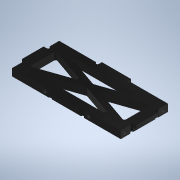
# Autodesk Inventor part: Trunk_horizontal_frame_04
Saved by Autodesk Inventor 2020.4 (Build 244396000, 396)
## iProperties
Created: 2016-05-21
Part Number: Trunk_horizontal_frame_04
Material: アセタール樹脂、黒
Document SubType Name: Modeling
Designer: hiroaki
Density: 1.425 g/cm^3
Appearance: 滑らか - 黒
Mass: 9.76521 g
Surface Area: 55.2384 cm^2
Volume: 6.85278 cm^3
Category: 胴体
d0: 1.050 mm
d1: 32.500 mm
d2: 75.000 mm
d3: 40.000 mm
d48: 26.500 mm
d52: 5.000 mm
d21: 32.500 mm
d23: 2.000 mm
d30: 2.000 mm
d34: 8.750 mm
d53: 20.000 mm
d54: 3.100 mm
d55: 5.000 mm
d56: 5.000 mm
d57: 0.00 deg
d58: 2.500 mm
d59: 0.00 deg
d60: 5.000 mm
d62: 2.500 mm
d66: 2.500 mm
d70: 2.500 mm
d74: 2.500 mm
Author: hiroaki
Autodesk Inventor part; units mm, degrees
ref_plane "YZ Plane" through (0, 0, 0) normal (1, 0, 0) x (0, 1, 0)
ref_plane "XZ Plane" through (0, 0, 0) normal (0, 1, 0) x (-1, 0, 0)
ref_plane "XY Plane" through (0, 0, 0) normal (0, 0, 1) x (1, 0, 0)
sketch "スケッチ1" plane through (0, 0, 0) normal (0, 0, 1) x (1, 0, 0)
  line L0 (-37.5, 9.6) -> (-37.5, 16.25)
  line L1 (-37.5, 16.25) -> (-20, 16.25)
  line L2 (20, 16.25) -> (37.5, 16.25)
  line L3 (37.5, 16.25) -> (37.5, 9.6)
  line L4 (0, 0) -> (0, 16.25) construction
  line L5 (0, 0) -> (39.5, 0) construction
  line L6 (37.5, 7.5) -> (39.5, 7.5)
  line L7 (39.5, 7.5) -> (39.5, -7.5)
  line L8 (39.5, -7.5) -> (37.5, -7.5)
  line L9 (-20, -16.25) -> (20, -16.25) construction
  line L10 (20, -16.25) -> (20, 16.25) construction
  line L11 (20, 16.25) -> (-20, 16.25) construction
  line L12 (-20, 16.25) -> (-20, -16.25) construction
  line L13 (-20, -16.25) -> (20, 16.25) construction
  line L14 (20, -16.25) -> (-20, 16.25) construction
  line L15 (-37.5, -16.25) -> (37.5, -16.25) construction
  line L16 (37.5, -16.25) -> (37.5, 16.25) construction
  line L17 (37.5, 16.25) -> (-37.5, 16.25) construction
  line L18 (-37.5, 16.25) -> (-37.5, -16.25) construction
  line L19 (-37.5, -16.25) -> (37.5, 16.25) construction
  line L20 (37.5, -16.25) -> (-37.5, 16.25) construction
  arc A0 (37.5, 9.6) -> (37.5, 7.5) centre (37.5, 8.55) ccw
  arc A1 (37.5, -7.5) -> (37.5, -9.6) centre (37.5, -8.55) ccw
  line L21 (37.5, -9.6) -> (37.5, -16.25)
  line L22 (37.5, -16.25) -> (20, -16.25)
  line L23 (20, -16.25) -> (12.1, -16.25)
  line L24 (-20, 16.25) -> (-12.1, 16.25)
  line L25 (-10, 16.25) -> (-10, 18.25)
  line L26 (-10, 18.25) -> (10, 18.25)
  line L27 (10, 18.25) -> (10, 16.25)
  line L28 (20, 16.25) -> (12.1, 16.25)
  arc A2 (-12.1, 16.25) -> (-10, 16.25) centre (-11.05, 16.25) ccw
  arc A3 (10, 16.25) -> (12.1, 16.25) centre (11.05, 16.25) ccw
  line L29 (-37.5, 7.5) -> (-39.5, 7.5)
  line L30 (-39.5, 7.5) -> (-39.5, -7.5)
  line L31 (-39.5, -7.5) -> (-37.5, -7.5)
  arc A4 (-37.5, 7.5) -> (-37.5, 9.6) centre (-37.5, 8.55) ccw
  arc A5 (-37.5, -9.6) -> (-37.5, -7.5) centre (-37.5, -8.55) ccw
  line L32 (-37.5, -9.6) -> (-37.5, -16.25)
  line L33 (-37.5, -16.25) -> (-20, -16.25)
  line L34 (-20, -16.25) -> (-12.1, -16.25)
  line L35 (-10, -16.25) -> (-10, -18.25)
  line L36 (-10, -18.25) -> (10, -18.25)
  line L37 (10, -18.25) -> (10, -16.25)
  arc A6 (-10, -16.25) -> (-12.1, -16.25) centre (-11.05, -16.25) ccw
  arc A7 (12.1, -16.25) -> (10, -16.25) centre (11.05, -16.25) ccw
  line L38 (-16.55, 19.1799) -> (-13.45, 19.1799) construction
  line L39 (-13.45, 19.1799) -> (-13.45, 12.4242) construction
  line L40 (-13.45, 12.4242) -> (-16.55, 12.4242) construction
  line L41 (-16.55, 12.4242) -> (-16.55, 19.1799) construction
  line L42 (-15, 19.1799) -> (-15, 12.4242) construction
  point P0 (0, 18.25)
  point P1 (0, 0)
  dimension "d0" = 1.05
  dimension "d1" = 32.5
  dimension "d2" = 75
  dimension "d3" = 40
  dimension "d23" = 2
  dimension "d30" = 2
  dimension "d34" = 8.75
  dimension "d53" = 20
  dimension "d54" = 3.1
  dimension "d55" = 5
  dimension "d85" = 32.5
  constraints: 86 end point, 17 point on line, 16 point on circle, 12 perpendicular, 9 midpoint, 8 centre point, 7 equal radius, 7 parallel, 6 horizontal, 6 symmetric about line, 5 tangent, 4 collinear, 2 vertical, 2 vertical alignment, 1 other
  measures "d0" radius of A0
  measures "d1" distance between parallel lines of L9 L11
  measures "d2" distance of L2.end L0.end
  measures "d3" distance between parallel lines of L10 L12
  measures "d23" distance of L6.start L6.end
  measures "d30" distance between parallel lines of L26 L11
  measures "d34" distance between parallel lines of L17 L29
  measures "d53" distance of L25.end L26.end
  measures "d54" distance of L38.start L38.end
  measures "d55" distance between parallel lines of L25 L42
  measures "d85" distance between parallel lines of L15 L17
extrude "押し出し1" add sketch "スケッチ1" along normal blind 5
sketch "スケッチ2" plane through (0, 0, 0) normal (0, 0, -1) x (-1, 0, 0)
  line L0 (37.5, 9.6) -> (37.5, 16.25) projected
  line L1 (-37.5, 16.25) -> (-37.5, 9.6) projected
  line L2 (-45.6427, 17.3125) -> (-37.5, 17.3125)
  line L3 (-37.5, 17.3125) -> (-37.5, -16.751)
  line L4 (-37.5, -16.751) -> (-45.6427, -16.751)
  line L5 (-45.6427, -16.751) -> (-45.6427, 17.3125)
  line L6 (37.5, 21.1805) -> (43.358, 21.1805)
  line L7 (43.358, 21.1805) -> (43.358, -13.6193)
  line L8 (43.358, -13.6193) -> (37.5, -13.6193)
  line L9 (37.5, -13.6193) -> (37.5, 21.1805)
  line L10 (-20, -16.25) -> (-12.1, -16.25)
  line L11 (-17.1371, 25.1848) -> (11.8342, 25.1848)
  line L12 (11.8342, 25.1848) -> (11.8342, 16.25)
  line L13 (11.8342, 16.25) -> (-17.1371, 16.25)
  line L14 (-17.1371, 16.25) -> (-17.1371, 25.1848)
  line L15 (-13.151, -21.5857) -> (17.7795, -21.5857)
  line L16 (17.7795, -21.5857) -> (17.7795, -16.25)
  line L17 (17.7795, -16.25) -> (-13.151, -16.25)
  line L18 (-13.151, -16.25) -> (-13.151, -21.5857)
  line L19 (-12.1, 16.25) -> (-37.5, 16.25)
  line L20 (-37.5, -16.25) -> (-12.1, -16.25)
  point P0 (0, 0)
  constraints: 38 end point, 8 parallel, 4 horizontal, 4 perpendicular, 3 collinear
extrude "押し出し2" cut sketch "スケッチ2" against normal blind 2.5
sketch "スケッチ3" plane through (12.1, 16.25, 0) normal (0, 1, 0) x (1, 0, 0)
  line L0 (-2.1, 0) -> (-2.1, -5) projected
  line L1 (-2.1, -5) -> (-22.1, -5) construction
  line L2 (-12.1, -5) -> (-12.1, 7.4607) construction
  line L3 (25.4, 0) -> (25.4, -5) projected
  point P0 (-12.1, 0)
  point P1 (2.9, -2.5)
  point P2 (-27.1, -2.5)
  point P3 (25.4, -2.5)
  dimension "d60" = 5
  constraints: 2 end point, 2 horizontal alignment, 2 midpoint, 1 symmetric about line, 1 vertical
  measures "d60" distance from line of L0 point (2.9, -2.5)
hole "穴1" at (15, 16.25, 2.5) at (-15, 16.25, 2.5) direction (0, -1, 0) diameter 2.459 depth 2.5 thread size "M3x0.5" class "6H" standard "ISO Metric profile"
mirror "ミラー1" about plane through (0, 0, 0) normal (0, 1, 0) of "穴1"
sketch "スケッチ4" plane through (37.5, -16.25, 5) normal (1, 0, 0) x (0, 0, -1)
  line L0 (5, 16.25) -> (0, 16.25) construction
  line L1 (0, 23.75) -> (0, 8.75) construction
  line L2 (5, 6.65) -> (0, 6.65) projected
  line L3 (5, 0) -> (0, 0) projected
  point P0 (2.5, 3)
  point P1 (2.5, 29.5)
  point P2 (2.5, 6.65)
  dimension "d86" = 3
  dimension "d87" = 26.5
  constraints: 2 end point, 2 midpoint, 2 vertical alignment, 1 symmetric about line
  measures "d86" distance from line of L3 point (2.5, 3)
  measures "d87" distance of point (2.5, 29.5) point (2.5, 3)
hole "穴2" at (37.5, -13.25, 2.5) at (37.5, 13.25, 2.5) direction (-1, 0, 0) diameter 2.459 depth 2.5 thread size "M3x0.5" class "6H" standard "ISO Metric profile"
mirror "ミラー2" about plane through (0, 0, 0) normal (1, 0, 0) of "穴2"
sketch "スケッチ5" plane through (0, 0, 0) normal (0, 0, -1) x (-1, 0, 0)
  line L0 (10, 16.25) -> (-10, 16.25) projected
  line L1 (-37.5, 7.5) -> (-37.5, 9.6) projected
  line L2 (-32.5, -11.25) -> (32.5, -11.25) construction
  line L3 (32.5, -11.25) -> (32.5, 11.25) construction
  line L4 (32.5, 11.25) -> (-32.5, 11.25) construction
  line L5 (-32.5, 11.25) -> (-32.5, -11.25) construction
  line L6 (-32.5, -11.25) -> (32.5, 11.25) construction
  line L7 (32.5, -11.25) -> (-32.5, 11.25) construction
  line L8 (-32.5, 9.1336) -> (-32.5, -9.1336)
  line L9 (-32.5, -9.1336) -> (-6.1141, 0)
  line L10 (-6.1141, 0) -> (-32.5, 9.1336)
  line L11 (-26.3859, 11.25) -> (26.3859, 11.25)
  line L12 (26.3859, 11.25) -> (0, 2.1164)
  line L13 (0, 2.1164) -> (-26.3859, 11.25)
  line L14 (-26.3859, -11.25) -> (26.3859, -11.25)
  line L15 (26.3859, -11.25) -> (0, -2.1164)
  line L16 (0, -2.1164) -> (-26.3859, -11.25)
  line L17 (32.5, 9.1336) -> (32.5, -9.1336)
  line L18 (32.5, -9.1336) -> (6.1141, 0)
  line L19 (6.1141, 0) -> (32.5, 9.1336)
  point P0 (-12.1, 16.25)
  point P1 (-20, 16.25)
  point P2 (-37.5, 16.25)
  point P3 (0, 0)
  dimension "d76" = 5
  dimension "d77" = 5
  dimension "d78" = 4
  dimension "d79" = 4
  dimension "d80" = 4
  dimension "d81" = 4
  constraints: 36 end point, 10 parallel, 4 collinear, 3 horizontal, 2 midpoint, 2 vertical, 1 perpendicular, 4 other
  measures "d76" distance between parallel lines of L4 L0
  measures "d77" distance between parallel lines of L1 L5
  measures "d78" distance between parallel lines of L19 L12
  measures "d79" distance between parallel lines of L15 L18
  measures "d80" distance between parallel lines of L10 L13
  measures "d81" distance between parallel lines of L16 L9
extrude "押し出し3" cut sketch "スケッチ5" against normal blind 10
fillet "フィレット1" radius 1.05 12 edges at (32.5, 9.1336, 2.5) (32.5, -9.1336, 2.5) (26.3859, 11.25, 2.5) (6.1141, 0, 2.5) (0, -2.1164, 2.5) (0, 2.1164, 2.5) (-32.5, -9.1336, 2.5) (26.3859, -11.25, 2.5) (-32.5, 9.1336, 2.5) (-26.3859, 11.25, 2.5) (-26.3859, -11.25, 2.5) (-6.1141, 0, 2.5)
equation "\"d85\" = d1"
equation "\"d60\" = d55"
equation "\"d77\" = d76"
equation "\"d79\" = d78"
equation "\"d80\" = d79"
equation "\"d81\" = d78"
equation "\"d48\" = 26.5"
equation "\"d52\" = 5"
